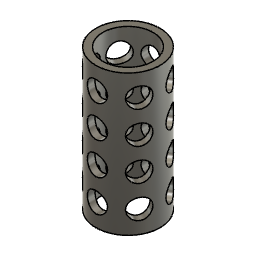
GasChargingCatridegCryoarmGuide v1 (Autodesk Fusion 360 design; units mm, degrees)
Autodesk Fusion 360 part; units mm, degrees
sketch "Skizze1" plane through (0, 0, 0) normal (0, 1, 0) x (1, 0, 0)
  circle A0 centre (0, 0) radius 8
  circle A1 centre (0, 0) radius 6.25
  dimension "d1" = 16
  dimension "d2" = 12.5
  constraint coincident A0.centre A1.centre
  measures "d1" diameter of A0
  measures "d2" diameter of A1
extrude "Extrusion1" add sketch "Skizze1" along normal blind 35
ref_plane "Arbeitsebene1" through (0, 24.3109, 8) normal (0, 0, 1) x (-1, 0, 0)
sketch "Skizze2" plane through (0, 24.3109, 8) normal (0, 0, 1) x (1, 0, 0)
  line L0 (0, 9.5) -> (0, -23.5) construction
  circle A0 centre (0, 5.1891) radius 2.5
  line L1 (8, 10.6891) -> (-8, 10.6891)
  circle A1 centre (0, -2.8109) radius 2.5
  circle A2 centre (0, -10.8109) radius 2.5
  circle A3 centre (0, -18.8109) radius 2.5
  line L2 (8, -24.3109) -> (-8, -24.3109)
  dimension "d6" = 5
  dimension "d7" = 5.5
  dimension "d10" = 8
  dimension "d11" = 0
  dimension "d12" = 5.5
  constraint vertical L0
  constraint coincident L0 A0.centre
  measures "d6" diameter of A0
  measures "d7" distance of A0.centre L1
  measures "d12" distance of A3.centre L2
extrude "Extrusion2" cut sketch "Skizze2" against normal through all
pattern_circular "C-Anordnung1" count 6 over 360 about axis through (0, 0, 0) along (0, 1, 0) of "Extrusion2"
